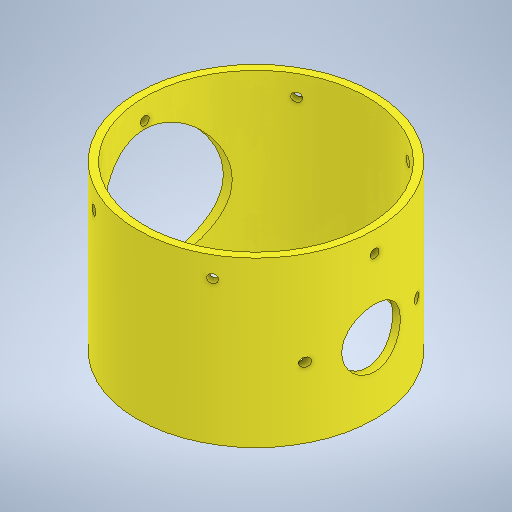
# Autodesk Inventor part: 130 part 1
Saved by Autodesk Inventor 2025.1 (Build 291241000, 241)
## iProperties
Created: 2024-08-01
Part Number: 130 part 1
Material: Aluminum 6061-AHC
Document SubType Name: Modeling
Designer: ffogue
Density: 2.7 g/cm^3
Appearance: Canary
Author: ffogue
Autodesk Inventor part; units mm, degrees
ref_plane "XZ Plane" through (0, 0, 0) normal (0, 1, 0) x (-1, 0, 0)
sketch "Sketch1" plane through (0, 0, 0) normal (0, 0, 1) x (1, 0, 0)
  circle A0 centre (0, 0) radius 40.5
  circle A1 centre (0, 0) radius 38
  dimension "d0" = 81
  dimension "d1" = 76
  constraints: 2 centre point, 2 coincident
  measures "d0" diameter of A0
  measures "d1" diameter of A1
extrude "Extrusion1" add sketch "Sketch1" against normal blind 56
ref_plane "Work Plane1" through (40.5, 0, 0) normal (1, 0, 0) x (0, 1, 0)
sketch "Sketch2" plane through (40.5, 0, 0) normal (1, 0, 0) x (0, 1, 0)
  line L0 (-40.5, -56) -> (40.5, -56) projected
  line L1 (40.5, 0) -> (-40.5, 0) projected
  line L2 (40.5, 0) -> (40.5, -56) projected
  line L3 (-40.5, 0) -> (-40.5, -56) projected
  point P0 (0, 0)
  point P1 (-19, -32)
  point P2 (19, -32)
  point P3 (0, 0)
  dimension "d5" = 24
  dimension "d6" = 19
  dimension "d7" = 19
  constraints: 1 horizontal alignment, 1 midpoint
  measures "d5" distance from line of L0 point (-19, -32)
  measures "d6" horizontal distance of point (-19, -32) point (0, 0)
  measures "d7" horizontal distance of point (0, 0) point (19, -32)
hole "Hole1" at (40.5, -19, -32) at (40.5, 19, -32) direction (-1, 0, 0) diameter 3 depth 9
sketch "Sketch3" plane through (40.5, 0, 0) normal (1, 0, 0) x (0, 1, 0)
  point P0 (0, 0)
  point P1 (0, -7)
  dimension "d15" = 7
  constraints: 1 vertical alignment
  measures "d15" distance of point (0, 0) point (0, -7)
hole "Hole2" at (40.5, 0, -7) direction (-1, 0, 0) diameter 3 depth 3
pattern_circular "Circular Pattern1" count 6 over 360 about axis through (0, 0, 0) along (0, 0, -1) of "Hole2"
sketch "Sketch5" plane through (40.5, 0, 0) normal (1, 0, 0) x (0, 1, 0)
  circle A0 centre (0, -32) radius 10
  line L0 (-40.5, -56) -> (40.5, -56) projected
  point P0 (0, 0)
  dimension "d33" = 20
  dimension "d34" = 24
  constraints: 1 centre point, 1 vertical alignment
  measures "d33" diameter of A0
  measures "d34" distance from line of L0 A0.centre
extrude "Extrusion4" cut sketch "Sketch5" against normal blind 4
ref_plane "Work Plane2" through (-40.5, 0, 0) normal (-1, 0, 0) x (0, -1, 0)
sketch "Sketch6" plane through (-40.5, 0, 0) normal (-1, 0, 0) x (0, -1, 0)
  circle A0 centre (0, -32) radius 22.5
  line L0 (-40.5, -56) -> (40.5, -56) projected
  point P0 (0, 0)
  dimension "d38" = 45
  dimension "d39" = 24
  constraints: 1 centre point, 1 vertical alignment
  measures "d38" diameter of A0
  measures "d39" distance from line of L0 A0.centre
extrude "Extrusion5" cut sketch "Sketch6" against normal up to surface
equation "\"d7\" = d6"
body "Solid1"
